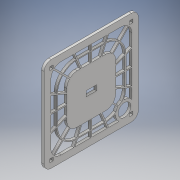
# Autodesk Inventor part: NewFront_F
Saved by Autodesk Inventor 2017 (Build 210142000, 142)
## iProperties
Created: 2019-07-06
Part Number: NewFront_F
Material: Generic
Document SubType Name: Modeling
Designer: DDeGo
Density: 1 g/cm^3
Appearance: Default
Author: DDeGo
Autodesk Inventor part; units mm, degrees
ref_plane "YZ Plane" through (0, 0, 0) normal (1, 0, 0) x (0, 1, 0)
ref_plane "XZ Plane" through (0, 0, 0) normal (0, 1, 0) x (-1, 0, 0)
ref_plane "XY Plane" through (0, 0, 0) normal (0, 0, 1) x (1, 0, 0)
sketch "Sketch1" plane through (0, 0, 0) normal (1, 0, 0) x (0, 1, 0)
  line L0 (0, 13.5) -> (156, 13.5)
  line L1 (169.5, 0) -> (169.5, -156)
  line L2 (156, -169.5) -> (0, -169.5)
  line L3 (-13.5, -156) -> (-13.5, 0)
  arc A0 (169.5, 0) -> (156, 13.5) centre (156, 0) ccw
  arc A1 (156, -169.5) -> (169.5, -156) centre (156, -156) ccw
  arc A2 (-13.5, -156) -> (0, -169.5) centre (0, -156) ccw
  arc A3 (0, 13.5) -> (-13.5, 0) centre (0, 0) ccw
  line L4 (19.5, 0.5) -> (136.5, 0.5)
  line L5 (156.5, -19.5) -> (156.5, -136.5)
  line L6 (136.5, -156.5) -> (19.5, -156.5)
  line L7 (-0.5, -136.5) -> (-0.5, -19.5)
  arc A4 (19.5, 0.5) -> (-0.5, -19.5) centre (19.5, -19.5) ccw
  arc A5 (-0.5, -136.5) -> (19.5, -156.5) centre (19.5, -136.5) ccw
  arc A6 (136.5, -156.5) -> (156.5, -136.5) centre (136.5, -136.5) ccw
  arc A7 (156.5, -19.5) -> (136.5, 0.5) centre (136.5, -19.5) ccw
  line L8 (156, 63.5) -> (0, 63.5)
  arc A8 (0, 63.5) -> (-63.5, 0) centre (0, 0) ccw
  line L9 (-63.5, 0) -> (-63.5, -156)
  arc A9 (-63.5, -156) -> (0, -219.5) centre (0, -156) ccw
  line L10 (0, -219.5) -> (156, -219.5)
  arc A10 (156, -219.5) -> (219.5, -156) centre (156, -156) ccw
  line L11 (219.5, -156) -> (219.5, 0)
  arc A11 (219.5, 0) -> (156, 63.5) centre (156, 0) ccw
  dimension "d0" = 13.5
  dimension "d1" = 183
  dimension "d2" = 183
  dimension "d15" = 13
  dimension "d16" = 13
  dimension "d17" = 13
  dimension "d18" = 13
  dimension "d19" = 20
  dimension "d41" = 50
  constraints: 24 end point, 24 point on circle, 16 tangent, 12 centre point, 6 equal radius, 6 parallel, 3 perpendicular, 2 horizontal, 8 other
  measures "d0" radius of A0
  measures "d1" distance between parallel lines of L2 L0
  measures "d2" distance between parallel lines of L1 L3
  measures "d15" distance between parallel lines of L3 L7
  measures "d16" distance between parallel lines of L0 L4
  measures "d17" distance between parallel lines of L1 L5
  measures "d18" distance between parallel lines of L2 L6
  measures "d19" radius of A4
  measures "d41" distance between parallel lines of L0 L8
extrude "Extrusion1" add sketch "Sketch1" along normal blind 5 contours L0 A0 L1 A1 L2 A2 L3 A3
sketch "Sketch3" plane through (5, 0, 0) normal (1, 0, 0) x (0, 0, -1)
  line L0 (105.5, 30.5) -> (50.5, 30.5)
  line L1 (30.5, 50.5) -> (30.5, 105.5)
  line L2 (50.5, 125.5) -> (105.5, 125.5)
  line L3 (125.5, 105.5) -> (125.5, 50.5)
  line L4 (125.5, 30.5) -> (30.5, 125.5) construction
  line L5 (30.5, 30.5) -> (125.5, 125.5) construction
  arc A0 (169.5, 156) -> (156, 169.5) centre (156, 156) ccw projected
  line L6 (0, 0) -> (156, 156) construction
  arc A1 (-0.5, 19.5) -> (19.5, -0.5) centre (19.5, 19.5) ccw projected
  line L7 (-0.5, 19.5) -> (-0.5, 136.5) projected
  arc A2 (19.5, 156.5) -> (-0.5, 136.5) centre (19.5, 136.5) ccw projected
  line L8 (19.5, 156.5) -> (136.5, 156.5) projected
  arc A3 (156.5, 136.5) -> (136.5, 156.5) centre (136.5, 136.5) ccw projected
  line L9 (156.5, 136.5) -> (156.5, 19.5) projected
  arc A4 (136.5, -0.5) -> (156.5, 19.5) centre (136.5, 19.5) ccw projected
  line L10 (136.5, -0.5) -> (19.5, -0.5) projected
  line L11 (156, 169.5) -> (0, 169.5) projected
  arc A5 (0, 169.5) -> (-13.5, 156) centre (0, 156) ccw projected
  line L12 (-13.5, 156) -> (-13.5, 0) projected
  arc A6 (-13.5, 0) -> (0, -13.5) centre (0, 0) ccw projected
  line L13 (0, -13.5) -> (156, -13.5) projected
  arc A7 (156, -13.5) -> (169.5, 0) centre (156, 0) ccw projected
  line L14 (169.5, 0) -> (169.5, 156) projected
  arc A8 (169.5, 156) -> (156, 169.5) centre (156, 156) ccw projected
  line L15 (30.5, 79.25) -> (-39.5, 79.25)
  line L16 (-39.5, 79.25) -> (-39.5, 76.75)
  line L17 (-39.5, 76.75) -> (30.5, 76.75)
  line L18 (30.5, 76.75) -> (30.5, 79.25)
  line L19 (30.5, 78) -> (78, 78) construction
  line L20 (34.5941, 58.6677) -> (33.6374, 60.9774)
  line L21 (-30.0775, 31.8798) -> (34.5941, 58.6677)
  line L22 (33.6374, 60.9774) -> (-31.0342, 34.1895)
  line L23 (-31.0342, 34.1895) -> (-30.0775, 31.8798)
  line L24 (45.2963, 43.5285) -> (43.5285, 45.2963)
  line L25 (-4.2012, -5.9689) -> (45.2963, 43.5285)
  line L26 (43.5285, 45.2963) -> (-5.9689, -4.2012)
  line L27 (-5.9689, -4.2012) -> (-4.2012, -5.9689)
  line L28 (60.9774, 33.6374) -> (58.6677, 34.5941)
  line L29 (34.1895, -31.0342) -> (60.9774, 33.6374)
  line L30 (58.6677, 34.5941) -> (31.8798, -30.0775)
  line L31 (31.8798, -30.0775) -> (34.1895, -31.0342)
  line L32 (79.25, 30.5) -> (76.75, 30.5)
  line L33 (79.25, -39.5) -> (79.25, 30.5)
  line L34 (76.75, 30.5) -> (76.75, -39.5)
  line L35 (76.75, -39.5) -> (79.25, -39.5)
  line L36 (97.3323, 34.5941) -> (95.0226, 33.6374)
  line L37 (124.1202, -30.0775) -> (97.3323, 34.5941)
  line L38 (95.0226, 33.6374) -> (121.8105, -31.0342)
  line L39 (121.8105, -31.0342) -> (124.1202, -30.0775)
  line L40 (112.4715, 45.2963) -> (110.7037, 43.5285)
  line L41 (161.9689, -4.2012) -> (112.4715, 45.2963)
  line L42 (110.7037, 43.5285) -> (160.2012, -5.9689)
  line L43 (160.2012, -5.9689) -> (161.9689, -4.2012)
  line L44 (122.3626, 60.9774) -> (121.4059, 58.6677)
  line L45 (187.0342, 34.1895) -> (122.3626, 60.9774)
  line L46 (121.4059, 58.6677) -> (186.0775, 31.8798)
  line L47 (186.0775, 31.8798) -> (187.0342, 34.1895)
  line L48 (125.5, 79.25) -> (125.5, 76.75)
  line L49 (195.5, 79.25) -> (125.5, 79.25)
  line L50 (125.5, 76.75) -> (195.5, 76.75)
  line L51 (195.5, 76.75) -> (195.5, 79.25)
  line L52 (121.4059, 97.3323) -> (122.3626, 95.0226)
  line L53 (186.0775, 124.1202) -> (121.4059, 97.3323)
  line L54 (122.3626, 95.0226) -> (187.0342, 121.8105)
  line L55 (187.0342, 121.8105) -> (186.0775, 124.1202)
  line L56 (110.7037, 112.4715) -> (112.4715, 110.7037)
  line L57 (160.2012, 161.9689) -> (110.7037, 112.4715)
  line L58 (112.4715, 110.7037) -> (161.9689, 160.2012)
  line L59 (161.9689, 160.2012) -> (160.2012, 161.9689)
  line L60 (95.0226, 122.3626) -> (97.3323, 121.4059)
  line L61 (121.8105, 187.0342) -> (95.0226, 122.3626)
  line L62 (97.3323, 121.4059) -> (124.1202, 186.0775)
  line L63 (124.1202, 186.0775) -> (121.8105, 187.0342)
  line L64 (76.75, 125.5) -> (79.25, 125.5)
  line L65 (76.75, 195.5) -> (76.75, 125.5)
  line L66 (79.25, 125.5) -> (79.25, 195.5)
  line L67 (79.25, 195.5) -> (76.75, 195.5)
  line L68 (58.6677, 121.4059) -> (60.9774, 122.3626)
  line L69 (31.8798, 186.0775) -> (58.6677, 121.4059)
  line L70 (60.9774, 122.3626) -> (34.1895, 187.0342)
  line L71 (34.1895, 187.0342) -> (31.8798, 186.0775)
  line L72 (43.5285, 110.7037) -> (45.2963, 112.4715)
  line L73 (-5.9689, 160.2012) -> (43.5285, 110.7037)
  line L74 (45.2963, 112.4715) -> (-4.2012, 161.9689)
  line L75 (-4.2012, 161.9689) -> (-5.9689, 160.2012)
  line L76 (33.6374, 95.0226) -> (34.5941, 97.3323)
  line L77 (-31.0342, 121.8105) -> (33.6374, 95.0226)
  line L78 (34.5941, 97.3323) -> (-30.0775, 124.1202)
  line L79 (-30.0775, 124.1202) -> (-31.0342, 121.8105)
  arc A9 (50.5, 125.5) -> (30.5, 105.5) centre (50.5, 105.5) ccw
  arc A10 (30.5, 50.5) -> (50.5, 30.5) centre (50.5, 50.5) ccw
  arc A11 (105.5, 30.5) -> (125.5, 50.5) centre (105.5, 50.5) ccw
  arc A12 (125.5, 105.5) -> (105.5, 125.5) centre (105.5, 105.5) ccw
  line L80 (10.5, 105.5) -> (10.5, 50.5)
  arc A13 (10.5, 50.5) -> (50.5, 10.5) centre (50.5, 50.5) ccw
  line L81 (50.5, 10.5) -> (105.5, 10.5)
  arc A14 (105.5, 10.5) -> (145.5, 50.5) centre (105.5, 50.5) ccw
  line L82 (145.5, 50.5) -> (145.5, 105.5)
  arc A15 (145.5, 105.5) -> (105.5, 145.5) centre (105.5, 105.5) ccw
  line L83 (105.5, 145.5) -> (50.5, 145.5)
  arc A16 (50.5, 145.5) -> (10.5, 105.5) centre (50.5, 105.5) ccw
  line L84 (12.5, 105.5) -> (12.5, 50.5)
  arc A17 (12.5, 50.5) -> (50.5, 12.5) centre (50.5, 50.5) ccw
  line L85 (50.5, 12.5) -> (105.5, 12.5)
  arc A18 (105.5, 12.5) -> (143.5, 50.5) centre (105.5, 50.5) ccw
  line L86 (143.5, 50.5) -> (143.5, 105.5)
  arc A19 (143.5, 105.5) -> (105.5, 143.5) centre (105.5, 105.5) ccw
  line L87 (105.5, 143.5) -> (50.5, 143.5)
  arc A20 (50.5, 143.5) -> (12.5, 105.5) centre (50.5, 105.5) ccw
  line L88 (83, 68) -> (73, 68)
  line L89 (73, 68) -> (73, 88)
  line L90 (73, 88) -> (83, 88)
  line L91 (83, 88) -> (83, 68)
  line L92 (83, 68) -> (73, 88) construction
  line L93 (73, 68) -> (83, 88) construction
  point P0 (34.1157, 59.8225)
  point P1 (44.4124, 44.4124)
  point P2 (59.8225, 34.1157)
  point P3 (78, 30.5)
  point P4 (96.1775, 34.1157)
  point P5 (111.5876, 44.4124)
  point P6 (121.8843, 59.8225)
  point P7 (125.5, 78)
  point P8 (121.8843, 96.1775)
  point P9 (111.5876, 111.5876)
  point P10 (96.1775, 121.8843)
  point P11 (78, 125.5)
  point P12 (59.8225, 121.8843)
  point P13 (44.4124, 111.5876)
  point P14 (34.1157, 96.1775)
  dimension "d28" = 95
  dimension "d29" = 95
  dimension "d30" = 2.5
  dimension "d31" = 70
  dimension "d34" = 360
  dimension "d38" = 20
  dimension "d39" = 2
  dimension "d40" = 11
  dimension "d44" = 10
  dimension "d45" = 20
  constraints: 172 end point, 24 point on circle, 12 centre point, 10 parallel, 9 point on line, 8 tangent, 6 midpoint, 5 perpendicular, 4 horizontal, 3 equal radius, 159 other
  measures "d28" distance of L4.end L5.end
  measures "d29" distance of L5.end L4.start
  measures "d30" distance of L15.end L16.end
  measures "d31" distance of L15.start L15.end
  measures "d38" radius of A9
  measures "d39" distance between parallel lines of L80 L84
  measures "d40" distance between parallel lines of L7 L80
  measures "d44" distance of L89.end L90.end
  measures "d45" distance of L88.end L89.end
extrude "Extrusion3" add sketch "Sketch3" against normal up to surface (5 mm away) contours L33 L85 L34 L0 | L0 L29 L28 L30 A10 L25 L24 L26 L1 L21 L20 L22 L77 L76 L78 A9 L73 L72 L74 L2 L69 L68 L70 L61 L60 L62 A12 L57 L56 L58 L3 L53 L52 L54 L45 L44 L46 A11 L41 L40 L42 L37 L36 L38 | L38 L36 L37 L0 | L0 L37 A18 L85 L38 | L85 L38 L81 L33 | L33 L81 L34 L85 | L29 L85 A17 L30 L0 | L0 L30 L28 L29 | L34 L81 L29 L85 | L85 A18 L37 A14 L81 L38 | L33 L10 L34 L81 | L29 L81 A13 L30 A17 L85 | A18 L42 A14 L37 | L81 A14 L37 L10 L38 | L33 L13 L34 L10 | L30 A13 L25 A17 | L29 L10 L30 A13 L81 | A11 L41 A18 L42 | L42 L40 L41 A11 | A18 L41 A14 L42 | L10 L37 L13 L38 | L33 L35 L34 L13 | A10 L26 L24 L25 | L25 A17 L26 A10 | L25 A13 L26 A17 | L29 L13 L30 L10 | A14 L41 A4 L42 | A18 L46 A14 L41 | L13 L37 L39 L38 | L25 A1 L26 A13 | L26 A13 L21 A17 | L29 L31 L30 L13 | A4 L41 L43 L42 | A18 L86 L45 L82 A14 L46 | L46 L3 L45 L86 A18 | L25 L27 L26 A1 | A17 L84 L22 L1 L21 | L21 A13 L80 L22 L84 A17 | L46 L44 L45 L3 | A14 L82 L45 L9 L46 | L1 L22 L20 L21 | L21 L7 L22 L80 A13 | L9 L45 L14 L46 | L86 L50 L82 L45 | L21 L12 L22 L7 | L22 L80 L17 L84 | L3 L49 L86 L50 | L14 L45 L47 L46 | L86 L49 L82 L50 | L17 L84 L15 L1 | L21 L23 L22 L12 | L17 L80 L15 L84 | L50 L82 L49 L9 | L9 L49 L14 L50 | L86 L54 L82 L49 | L17 L12 L15 L7 | L7 L15 L80 L17 | L15 L80 L77 L84 | L54 L52 L53 L3 | L3 L53 A19 L86 L54 | L14 L49 L51 L50 | L86 A19 L53 A15 L82 L54 | L77 L84 A20 L78 L1 | L1 L78 L76 L77 | L17 L16 L15 L12 | L77 L80 A16 L78 A20 L84 | L54 L82 A15 L53 L9 | L9 L53 L14 L54 | L77 L12 L78 L7 | L7 L78 A16 L80 L77 | A19 L58 A15 L53 | L14 L53 L55 L54 | L78 A16 L73 A20 | L77 L79 L78 L12 | L58 L56 L57 A12 | A19 L57 A15 L58 | A9 L74 L72 L73 | L73 A20 L74 A9 | L73 A16 L74 A20 | A19 L62 A15 L57 | L73 A2 L74 A16 | L74 A16 L69 A20 | L73 L75 L74 A2 | A19 L87 L61 L83 A15 L62 | L62 L2 L61 L87 A19 | A20 L87 L70 L2 L69 | L69 A16 L83 L70 L87 A20 | L62 L60 L61 L2 | A15 L83 L61 L8 L62 | L62 L8 L61 L11 | L11 L61 L63 L62 | L2 L70 L68 L69 | L69 L8 L70 L83 A16 | L69 L71 L70 L11 | L11 L70 L8 L69 | L87 L66 L83 L61 | L70 L83 L65 L87 | L2 L65 L87 L66 | L87 L65 L83 L66 | L66 L8 L65 L11 | L11 L65 L67 L66 | L66 L83 L65 L8
extrude "Extrusion4" cut sketch "Sketch1" along normal blind 10 contours A11 L11 A10 L10 A9 L9 A8 L8
sketch "Sketch4" plane through (0, 0, 0) normal (-1, 0, 0) x (0, 0, 1)
  circle A0 centre (-142.5, 142.5) radius 12.5
  circle A1 centre (-142.5, 142.5) radius 17.5
  line L0 (-156, 169.5) -> (0, 169.5) projected
  line L1 (-169.5, 0) -> (-169.5, 156) projected
  line L2 (-111.8688, 156.5) -> (-136.5, 156.5) projected
  arc A2 (-106.4788, 143.4874) -> (-143.4874, 106.4788) centre (-105.5, 105.5) ccw projected
  line L3 (-131.6536, 133.0679) -> (-133.0679, 131.6536)
  line L4 (-133.0679, 131.6536) -> (-120.3316, 118.9173)
  line L5 (-120.3316, 118.9173) -> (-118.9173, 120.3316)
  line L6 (-118.9173, 120.3316) -> (-131.6536, 133.0679)
  arc A3 (-105.5, 125.5) -> (-125.5, 105.5) centre (-105.5, 105.5) ccw projected
  arc A4 (-105.5, 125.5) -> (-125.5, 105.5) centre (-105.5, 105.5) ccw projected
  line L7 (-119.6244, 119.6244) -> (-105.5, 105.5) construction
  line L8 (-125.5, 105.5) -> (-125.5, 99.0281) projected
  point P0 (0, 0)
  point P1 (-105.5, 141)
  point P2 (-141, 105.5)
  dimension "d46" = 27
  dimension "d47" = 27
  dimension "d48" = 5
  dimension "d52" = 45
  dimension "d53" = 2
  dimension "d61" = 25
  constraints: 10 end point, 2 centre point, 2 parallel, 1 coincident, 1 midpoint, 1 perpendicular, 1 point on circle, 3 other
  measures "d46" distance from line of L0 A0.centre
  measures "d47" distance from line of L1 A0.centre
  measures "d48" radial gap between concentric circles of A1 A0
  measures "d52" angle of L8 L7
  measures "d53" distance between parallel lines of L6 L4
  measures "d61" diameter of A0
extrude "Extrusion5" add sketch "Sketch4" against normal up to surface (5 mm away)
fillet "Fillet1" radius 1.5 2 edges at (2.5, 140.3506, -125.1325) (2.5, 125.1325, -140.3506)
sketch "Sketch5" plane through (0, 0, 0) normal (-1, 0, 0) x (0, 0, 1)
  line L0 (-0.5, 0.5) -> (-155.5, 0.5) construction
  line L1 (-155.5, 0.5) -> (-155.5, 155.5) construction
  line L2 (-155.5, 155.5) -> (-0.5, 155.5) construction
  line L3 (-0.5, 155.5) -> (-0.5, 0.5) construction
  line L4 (-3.625, 158.625) -> (2.625, 158.625)
  line L5 (2.625, 158.625) -> (2.625, 152.375)
  line L6 (2.625, 152.375) -> (-3.625, 152.375)
  line L7 (-3.625, 152.375) -> (-3.625, 158.625)
  line L8 (-3.625, 158.625) -> (2.625, 152.375) construction
  line L9 (2.625, 158.625) -> (-3.625, 152.375) construction
  line L10 (-3.625, 3.625) -> (2.625, 3.625)
  line L11 (2.625, 3.625) -> (2.625, -2.625)
  line L12 (2.625, -2.625) -> (-3.625, -2.625)
  line L13 (-3.625, -2.625) -> (-3.625, 3.625)
  line L14 (-3.625, 3.625) -> (2.625, -2.625) construction
  line L15 (2.625, 3.625) -> (-3.625, -2.625) construction
  line L16 (-158.625, 3.625) -> (-152.375, 3.625)
  line L17 (-152.375, 3.625) -> (-152.375, -2.625)
  line L18 (-152.375, -2.625) -> (-158.625, -2.625)
  line L19 (-158.625, -2.625) -> (-158.625, 3.625)
  line L20 (-158.625, 3.625) -> (-152.375, -2.625) construction
  line L21 (-152.375, 3.625) -> (-158.625, -2.625) construction
  line L22 (-152.375, 152.375) -> (-158.625, 152.375)
  line L23 (-158.625, 152.375) -> (-158.625, 158.625)
  line L24 (-158.625, 158.625) -> (-152.375, 158.625)
  line L25 (-152.375, 158.625) -> (-152.375, 152.375)
  line L26 (-152.375, 152.375) -> (-158.625, 158.625) construction
  line L27 (-158.625, 152.375) -> (-152.375, 158.625) construction
  line L28 (-156, -13.5) -> (0, -13.5) projected
  line L29 (-169.5, 156) -> (-169.5, 0) projected
  line L30 (13.5, 0) -> (13.5, 156) projected
  line L31 (0, 169.5) -> (-156, 169.5) projected
  point P0 (0, 0)
  dimension "d54" = 6.25
  dimension "d55" = 14
  dimension "d56" = 14
  dimension "d57" = 14
  dimension "d58" = 14
  constraints: 56 end point, 10 parallel, 8 midpoint, 7 equal length, 5 horizontal, 5 perpendicular
  measures "d54" distance of L4.start L4.end
  measures "d55" distance between parallel lines of L28 L0
  measures "d56" distance between parallel lines of L29 L1
  measures "d57" distance between parallel lines of L30 L3
  measures "d58" distance between parallel lines of L31 L2
extrude "Extrusion6" cut sketch "Sketch5" against normal blind 10
sketch "Sketch6" plane through (5, 0, 0) normal (1, 0, 0) x (0, 0, -1)
  arc A0 (144.4685, 154.844) -> (132.4701, 135.04) centre (142.5, 142.5) ccw projected
  circle A1 centre (142.5, 142.5) radius 12.5
  point P0 (0, 0)
  constraints: 1 centre point, 1 coincident, 1 concentric
extrude "Extrusion7" cut sketch "Sketch6" against normal blind 10
equation "\"d16\" = d15"
equation "\"d17\" = d15"
equation "\"d18\" = d15"
equation "\"d29\" = d28"
equation "\"d56\" = d55"
equation "\"d57\" = d55"
equation "\"d58\" = d55"
body "Solid1"
